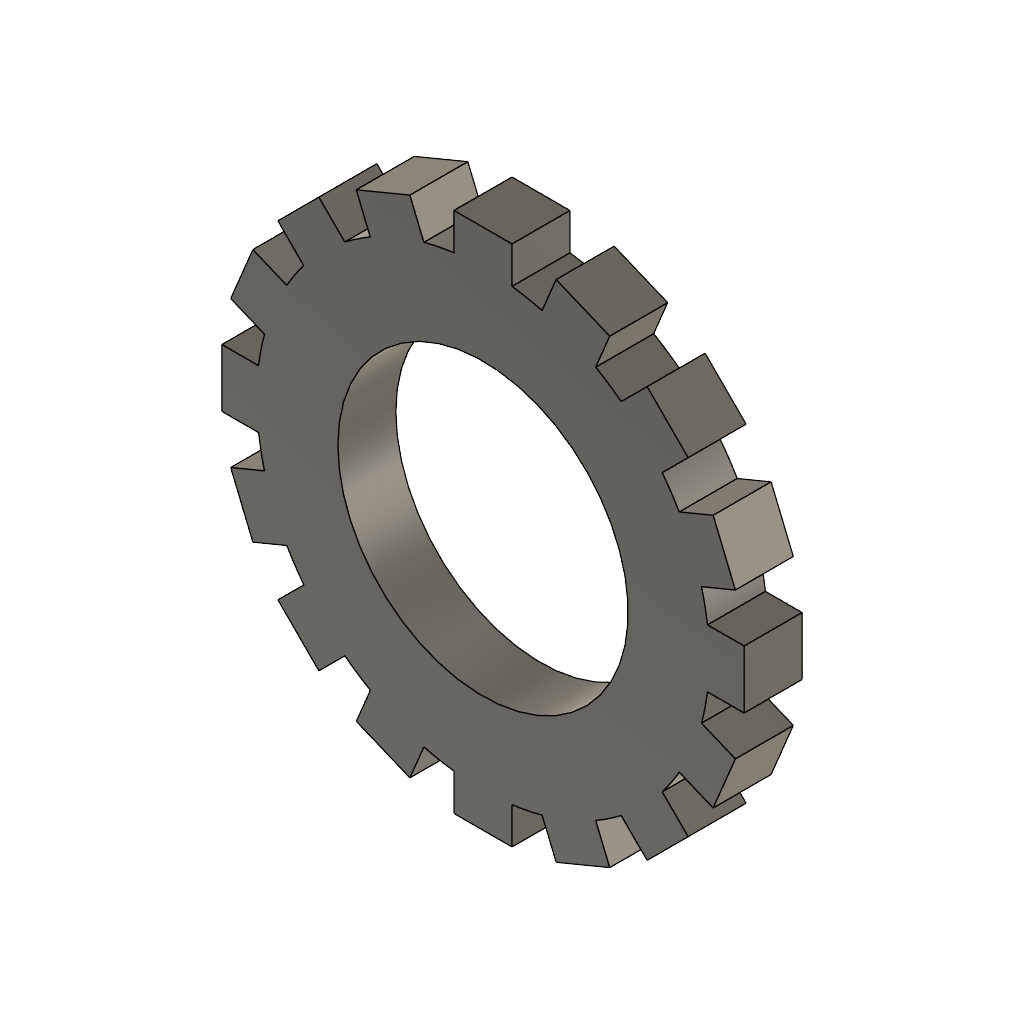
exercise 9 (Autodesk Fusion 360 design; units mm, degrees)
part number: 2026-10-06-22-01-51-755
Autodesk Fusion 360 part; units mm, degrees
sketch "Sketch1" plane through (0, 0, 0) normal (0, 1, 0) x (1, 0, 0)
  circle A0 centre (0, 0) radius 25
  line L0 (0, 0) -> (0, -50) construction
  line L1 (0, -45) -> (-5, -45)
  line L2 (-5, -45) -> (-5, -38.6782)
  line L3 (5, -45) -> (5, -38.6782)
  line L4 (0, -45) -> (5, -45)
  line L5 (12.6014, -43.488) -> (10.1821, -37.6474)
  line L6 (17.2208, -41.5746) -> (12.6014, -43.488)
  line L7 (17.2208, -41.5746) -> (21.8402, -39.6612)
  line L8 (21.8402, -39.6612) -> (19.4209, -33.8205)
  line L9 (28.2843, -35.3553) -> (23.8141, -30.8851)
  line L10 (31.8198, -31.8198) -> (28.2843, -35.3553)
  line L11 (31.8198, -31.8198) -> (35.3553, -28.2843)
  line L12 (35.3553, -28.2843) -> (30.8851, -23.8141)
  line L13 (39.6612, -21.8402) -> (33.8205, -19.4209)
  line L14 (41.5746, -17.2208) -> (39.6612, -21.8402)
  line L15 (41.5746, -17.2208) -> (43.488, -12.6014)
  line L16 (43.488, -12.6014) -> (37.6474, -10.1821)
  line L17 (45, -5) -> (38.6782, -5)
  line L18 (45, 0) -> (45, -5)
  line L19 (45, 0) -> (45, 5)
  line L20 (45, 5) -> (38.6782, 5)
  line L21 (43.488, 12.6014) -> (37.6474, 10.1821)
  line L22 (41.5746, 17.2208) -> (43.488, 12.6014)
  line L23 (41.5746, 17.2208) -> (39.6612, 21.8402)
  line L24 (39.6612, 21.8402) -> (33.8205, 19.4209)
  line L25 (35.3553, 28.2843) -> (30.8851, 23.8141)
  line L26 (31.8198, 31.8198) -> (35.3553, 28.2843)
  line L27 (31.8198, 31.8198) -> (28.2843, 35.3553)
  line L28 (28.2843, 35.3553) -> (23.8141, 30.8851)
  line L29 (21.8402, 39.6612) -> (19.4209, 33.8205)
  line L30 (17.2208, 41.5746) -> (21.8402, 39.6612)
  line L31 (17.2208, 41.5746) -> (12.6014, 43.488)
  line L32 (12.6014, 43.488) -> (10.1821, 37.6474)
  line L33 (5, 45) -> (5, 38.6782)
  line L34 (0, 45) -> (5, 45)
  line L35 (0, 45) -> (-5, 45)
  line L36 (-5, 45) -> (-5, 38.6782)
  line L37 (-12.6014, 43.488) -> (-10.1821, 37.6474)
  line L38 (-17.2208, 41.5746) -> (-12.6014, 43.488)
  line L39 (-17.2208, 41.5746) -> (-21.8402, 39.6612)
  line L40 (-21.8402, 39.6612) -> (-19.4209, 33.8205)
  line L41 (-28.2843, 35.3553) -> (-23.8141, 30.8851)
  line L42 (-31.8198, 31.8198) -> (-28.2843, 35.3553)
  line L43 (-31.8198, 31.8198) -> (-35.3553, 28.2843)
  line L44 (-35.3553, 28.2843) -> (-30.8851, 23.8141)
  line L45 (-39.6612, 21.8402) -> (-33.8205, 19.4209)
  line L46 (-41.5746, 17.2208) -> (-39.6612, 21.8402)
  line L47 (-41.5746, 17.2208) -> (-43.488, 12.6014)
  line L48 (-43.488, 12.6014) -> (-37.6474, 10.1821)
  line L49 (-45, 5) -> (-38.6782, 5)
  line L50 (-45, 0) -> (-45, 5)
  line L51 (-45, 0) -> (-45, -5)
  line L52 (-45, -5) -> (-38.6782, -5)
  line L53 (-43.488, -12.6014) -> (-37.6474, -10.1821)
  line L54 (-41.5746, -17.2208) -> (-43.488, -12.6014)
  line L55 (-41.5746, -17.2208) -> (-39.6612, -21.8402)
  line L56 (-39.6612, -21.8402) -> (-33.8205, -19.4209)
  line L57 (-35.3553, -28.2843) -> (-30.8851, -23.8141)
  line L58 (-31.8198, -31.8198) -> (-35.3553, -28.2843)
  line L59 (-31.8198, -31.8198) -> (-28.2843, -35.3553)
  line L60 (-28.2843, -35.3553) -> (-23.8141, -30.8851)
  line L61 (-21.8402, -39.6612) -> (-19.4209, -33.8205)
  line L62 (-17.2208, -41.5746) -> (-21.8402, -39.6612)
  line L63 (-17.2208, -41.5746) -> (-12.6014, -43.488)
  line L64 (-12.6014, -43.488) -> (-10.1821, -37.6474)
  arc A1 (-10.1821, -37.6474) -> (-5, -38.6782) centre (0, 0) ccw
  arc A2 (-23.8141, -30.8851) -> (-19.4209, -33.8205) centre (0, 0) ccw
  arc A3 (-33.8205, -19.4209) -> (-30.8851, -23.8141) centre (0, 0) ccw
  arc A4 (-38.6782, -5) -> (-37.6474, -10.1821) centre (0, 0) ccw
  arc A5 (-37.6474, 10.1821) -> (-38.6782, 5) centre (0, 0) ccw
  arc A6 (-30.8851, 23.8141) -> (-33.8205, 19.4209) centre (0, 0) ccw
  arc A7 (-19.4209, 33.8205) -> (-23.8141, 30.8851) centre (0, 0) ccw
  arc A8 (-5, 38.6782) -> (-10.1821, 37.6474) centre (0, 0) ccw
  arc A9 (10.1821, 37.6474) -> (5, 38.6782) centre (0, 0) ccw
  arc A10 (23.8141, 30.8851) -> (19.4209, 33.8205) centre (0, 0) ccw
  arc A11 (38.6782, 5) -> (37.6474, 10.1821) centre (0, 0) ccw
  arc A12 (33.8205, 19.4209) -> (30.8851, 23.8141) centre (0, 0) ccw
  arc A13 (37.6474, -10.1821) -> (38.6782, -5) centre (0, 0) ccw
  arc A14 (30.8851, -23.8141) -> (33.8205, -19.4209) centre (0, 0) ccw
  arc A15 (5, -38.6782) -> (10.1821, -37.6474) centre (0, 0) ccw
  arc A16 (19.4209, -33.8205) -> (23.8141, -30.8851) centre (0, 0) ccw
  dimension "d1" = 50
  dimension "d2" = 78
  dimension "d4" = 5
  constraint coincident A0.centre L0.start
  constraint vertical L0
  constraint coincident L0 L1.start
  constraint perpendicular L0 L1
  constraint perpendicular L1 L2
  constraint symmetric L0 L1.start L4.start
  constraint symmetric L0 L1.end L3.start
  constraint symmetric L0 L2.end L3.end
  constraint concentric A1 A15
  constraint concentric A2 A3
  constraint concentric A3 A4
  constraint concentric A4 A5
  constraint concentric A5 A6
  constraint concentric A11 A13
  constraint concentric A6 A7
  constraint concentric A7 A8
  constraint concentric A8 A9
  constraint concentric A9 A10
  constraint concentric A10 A12
  constraint concentric A11 A12
  constraint concentric A13 A14
  constraint concentric A14 A16
  constraint concentric A15 A16
  measures "d1" diameter of A0
  measures "d2" diameter of A15
  measures "d4" distance of L1.start L1.end
extrude "Extrude1" add sketch "Sketch1" along normal blind 10
